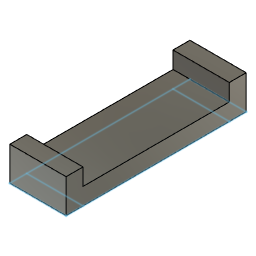
test-fit-weights (Autodesk Fusion 360 design; units mm, degrees)
Autodesk Fusion 360 part; units mm, degrees
sketch "Esquisse1" plane through (0, 0, 0) normal (0, 0, 1) x (1, 0, 0)
  line L0 (-78.1104, -5.5435) -> (-68.1104, -5.5435)
  line L1 (-68.1104, -5.5435) -> (-68.1104, -37.5435)
  line L2 (-68.1104, -37.5435) -> (-78.1104, -37.5435)
  line L3 (-78.1104, -37.5435) -> (-78.1104, -5.5435)
  line L4 (-78.1104, -8.5435) -> (-68.1104, -8.5435)
  line L5 (-78.1104, -34.5435) -> (-68.1104, -34.5435)
  dimension "d1" = 3
  dimension "d2" = 10
  dimension "d3" = 3
  dimension "d4" = 26
  constraint horizontal L0
  constraint vertical L1
  constraint horizontal L2
  constraint vertical L3
  constraint coincident L3 L4.start
  constraint coincident L1 L4.end
  constraint perpendicular L1 L4
  constraint coincident L3 L5.start
  constraint coincident L1 L5.end
  constraint perpendicular L1 L5
  measures "d1" distance of L0 L4
  measures "d2" distance of L5.start L5.end
  measures "d3" distance of L2 L5
  measures "d4" distance of L4 L5
extrude "Extrusion1" add sketch "Esquisse1" along normal blind 3
extrude "Extrusion2" add sketch "Esquisse1" along normal blind 6 contours L0 L1 L3 L4 | L1 L2 L3 L5
